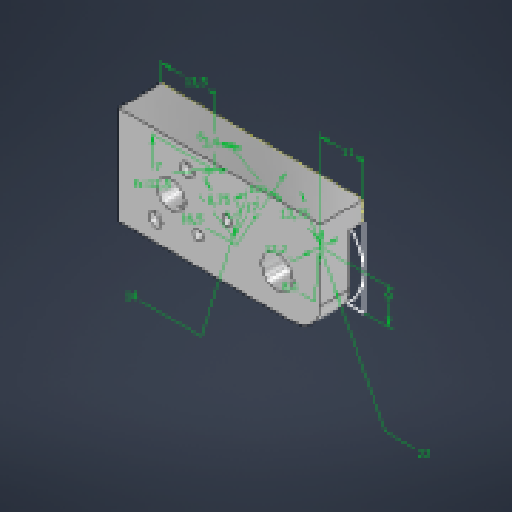
# Autodesk Inventor part: MocowaniePrzekladni
Saved by Autodesk Inventor 2023 (Build 270158000, 158)
## iProperties
Created: 2024-02-25
Part Number: MocowaniePrzekladni
Material: Aluminum 6061
Document SubType Name: Modeling
Designer: Michał
Density: 2.7 g/cm^3
Appearance: Aluminum - Flat
Author: Michał
## iProperties of the stored document MocowaniePrzekladni_3DPrint.ipt
Created: 2024-04-24
Part Number: MocowaniePrzekladni_3DPrint
Material: Generic
Document SubType Name: Modeling
Designer: Michał
Density: 1 g/cm^3
Appearance: Default
Author: Michał
Autodesk Inventor part; units mm, degrees
ref_plane "YZ Plane" through (0, 0, 0) normal (1, 0, 0) x (0, 1, 0)
ref_plane "XZ Plane" through (0, 0, 0) normal (0, 1, 0) x (-1, 0, 0)
ref_plane "XY Plane" through (0, 0, 0) normal (0, 0, 1) x (1, 0, 0)
sketch "Sketch1" plane through (0, 0, 0) normal (0, 0, 1) x (1, 0, 0)
  line L0 (51.5, 25) -> (0, 25)
  line L1 (0, 25) -> (0, 0)
  line L2 (0, 0) -> (51.5, 0)
  line L3 (51.5, 0) -> (51.5, 25)
  point P0 (0, 12.5)
  dimension "d85" = 25
  dimension "d86" = 51.5
  constraints: 8 end point, 2 parallel, 1 coincident, 1 horizontal, 1 midpoint, 1 perpendicular
  measures "d85" distance between parallel lines of L2 L0
  measures "d86" distance from line of point (0, 12.5) L3
extrude "Bryla" add sketch "Sketch1" along normal blind 11
sketch "Sketch3" plane through (0, 0, 0) normal (0, 0, -1) x (-1, 0, 0)
  circle A0 centre (-13.5, 12.5) radius 3.5
  circle A1 centre (-20.3053, 7) radius 7
  circle A2 centre (-27.6215, 13.8172) radius 8.25
  circle A3 centre (-40.5, 9) radius 11
  circle A4 centre (-40.5, 9) radius 4.05
  circle A5 centre (-40.5, 9) radius 6.1
  line L0 (-13.5, 12.5) -> (-20.3053, 7) construction
  line L1 (-20.3053, 7) -> (-27.6215, 13.8172) construction
  line L2 (-27.6215, 13.8172) -> (-40.5, 9) construction
  line L3 (-17.5442, 19.9762) -> (-9.4558, 5.0238) construction
  circle A6 centre (-9.4558, 5.0238) radius 1.7
  circle A7 centre (-17.5442, 19.9762) radius 1.7
  circle A8 centre (-17.5442, 19.9762) radius 3
  circle A9 centre (-9.4558, 5.0238) radius 3
  line L4 (0, 0) -> (-51.5, 0) construction
  line L5 (-40.5, 20) -> (-51.5, 20)
  line L6 (-51.5, 20) -> (-51.5, 0)
  line L7 (0, 0) -> (-51.5, 0)
  line L8 (-46.8246, 0) -> (-51.5, 0)
  line L9 (-34.1754, 0) -> (-29.5, 0)
  line L10 (-29.5, 0) -> (-29.5, 9)
  line L11 (-27.3053, 7) -> (-27.3053, 0)
  line L12 (-13.3053, 7) -> (-13.3053, 0)
  line L13 (-29.5, 0) -> (-27.3053, 0)
  line L14 (-35.8715, 13.8172) -> (-35.8715, 0)
  line L15 (-51.5, 0) -> (0, 0) construction
  line L16 (0, 0) -> (0, 25) construction
  line L17 (0, 0) -> (-51.5, 0) construction
  line L18 (0, 25) -> (0, 0) construction
  line L19 (0, 25) -> (0, 0) construction
  line L20 (0, 0) -> (-51.5, 0) construction
  line L21 (-51.5, 25) -> (0, 25) construction
  line L22 (-51.5, 0) -> (-51.5, 25) construction
  line L23 (0, 0) -> (-51.5, 0) construction
  line L24 (0, 0) -> (-51.5, 0) construction
  point P0 (-34.4011, 9.1163)
  point P1 (-35.822, 12.9148)
  point P2 (-27.1598, 5.5801)
  point P3 (-22.8938, 18.8508)
  point P4 (-29.9455, 5.9013)
  point P5 (-23.4992, 20.9635)
  point P6 (-19.82, 16.5003)
  point P7 (-34.57, 18.2647)
  point P8 (-20.5208, 12.676)
  point P9 (-19.3723, 13.9375)
  point P10 (-23.9846, 12.9551)
  point P11 (-16.7322, 13.0194)
  point P12 (-1.1315, 7.6691)
  point P13 (-16.5069, 14.2913)
  point P14 (-10.2995, 13.9166)
  point P15 (-16.9412, 13.1386)
  point P16 (-6.1553, 9.4162)
  point P17 (-15.1313, 21.7589)
  point P18 (-16.1793, 22.6477)
  point P19 (-13.5975, 9.0014)
  point P20 (-29.5, 0)
  point P21 (-27.6754, 0)
  point P22 (-20.3053, 0)
  point P23 (-34.1754, 0)
  point P24 (-27.3053, 5.5733)
  point P25 (-29.5, 5.7839)
  point P26 (-51.5, 9)
  dimension "d20" = 7
  dimension "d21" = 14
  dimension "d22" = 16.5
  dimension "d23" = 22
  dimension "d24" = 12.2
  dimension "d25" = 8.1
  dimension "d26" = 8.75
  dimension "d27" = 10
  dimension "d28" = 13.75
  dimension "d59" = 6
  dimension "d60" = 3.4
  dimension "d61" = 17
  dimension "d66" = 12.5
  dimension "d69" = 9
  dimension "d83" = 13.5
  dimension "d87" = 11
  constraints: 42 end point, 16 point on circle, 9 centre point, 7 coincident, 7 perpendicular, 6 tangent, 4 point on line, 2 vertical, 1 collinear, 1 equal radius, 1 horizontal, 1 midpoint, 7 other
  measures "d20" diameter of A0
  measures "d21" diameter of A1
  measures "d22" diameter of A2
  measures "d23" diameter of A3
  measures "d24" diameter of A5
  measures "d25" diameter of A4
  measures "d26" distance of L0.start L0.end
  measures "d27" distance of L0.end L1.end
  measures "d28" distance of L1.end L2.end
  measures "d59" diameter of A8
  measures "d60" diameter of A7
  measures "d61" distance of L3.start L3.end
  measures "d66" distance from line of L4 L0.start
  measures "d69" distance from line of L4 A3.centre
  measures "d83" distance from line of L0.start L16
  measures "d87" distance from line of L22 A3.centre
extrude "Przelot" cut sketch "Sketch3" against normal through all contours A0 A1 | A1 A0 | A4 | A6 | A7
extrude "kolo3" cut sketch "Sketch3" against normal blind 3.5 contours A1 A0 | A3 A2 A5 | A2 L14 A5 L7 A3 | L11 L7 L10 A2 | A2 A5 L14 | L10 A2 A3 | A3 L6 L5 | L10 L7 A3 A2 | A5 A2 | A2 A5 L14 | L14 A5 | A3 L7 L14 A5 A2 | A3 L7 L6 | A3 L7 | A4 picked at (-14.968, 10.5481)
extrude "kolo1" cut sketch "Sketch3" against normal blind 9.3 contours A0 A1 | A1 A0 | A0 A1 A2 | A2 A1 | L12 L7 A1 | A1 A2 L11 | L7 L11 A2 A1
extrude "kolo2" cut sketch "Sketch3" against normal blind 6 contours A2 A1 | A1 L11 A2 L10 A3 | A1 A2 L11 | A3 A2 A5 | L10 A2 A3 | A5 A2
hole "osieMale" at (27.6215, 13.8172, 0) at (20.3053, 7, 0) direction (0, 0, 1) diameter 2.5 end through all
extrude "kolnierzLozyska" cut sketch "Sketch3" against normal blind 1 from surface at -3.5 contours A2 A5 L14 | L14 A5 picked at (-35.5053, 8.9668)
extrude "lbySrob" cut sketch "Sketch3" against normal up to surface (9.3 mm away) contours A6 | A7 | A8 | A9
fillet "Fillet1" radius 7 1 edges at (51.5, 0, 7.25)
body "Solid1"
